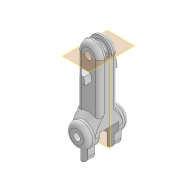
# Autodesk Inventor part: ring_f2
Saved by Autodesk Inventor 2020.2 (Build 242310000, 310)
## iProperties
Created: 2020-04-08
Part Number: ring_f2
Material: Generic
Document SubType Name: Modeling
Designer: Bardo91
Density: 1 g/cm^3
Appearance: Default
Author: Bardo91
Autodesk Inventor part; units mm, degrees
ref_plane "YZ Plane" through (0, 0, 0) normal (1, 0, 0) x (0, 1, 0)
ref_plane "XY Plane" through (0, 0, 0) normal (0, 0, 1) x (1, 0, 0)
sketch "Sketch1" plane through (0, 0, 0) normal (0, 0, 1) x (1, 0, 0)
  circle A0 centre (0, 0) radius 1.5
  circle A1 centre (0, 0) radius 5
  line L0 (0, 0) -> (0, 28)
  circle A2 centre (0, 28) radius 1.5
  circle A3 centre (0, 28) radius 5
  line L1 (-5, 28) -> (-5, 0)
  line L2 (5, 28) -> (5, 0)
  dimension "d0" = 3
  dimension "d1" = 10
  dimension "d2" = 28
  dimension "d3" = 3
  dimension "d4" = 10
  constraints: 6 end point, 4 centre point, 4 coincident, 4 point on circle, 3 tangent, 1 vertical
  measures "d0" diameter of A0
  measures "d1" diameter of A1
  measures "d2" distance of L0.start L0.end
  measures "d3" diameter of A2
  measures "d4" diameter of A3
extrude "base" add sketch "Sketch1" along normal blind 8
sketch "Sketch2" plane through (0, 0, 8) normal (0, 0, 1) x (1, 0, 0)
  circle A0 centre (0, 0) radius 1.5
  circle A1 centre (0, 0) radius 5
  dimension "d29" = 3.5
  dimension "d7" = 3
  dimension "d8" = 10
  constraints: 2 centre point, 2 coincident
  measures "d7" diameter of A0
  measures "d8" diameter of A1
extrude "joint" add sketch "Sketch2" along normal blind 5
ref_plane "Work Plane1" through (0, 0, 4) normal (0, 0, 1) x (1, 0, 0)
mirror "Mirror1" about plane through (0, 0, 4) normal (0, 0, 1) of "joint"
chamfer "Chamfer1" distance 2 angle 45 2 edges at (0, 5, 8) (0, 5, 0)
sketch "Sketch3" plane through (0, 0, 4) normal (0, 0, 1) x (1, 0, 0)
  circle A0 centre (0, 0) radius 1.5 projected
  circle A1 centre (0, 0) radius 5.25
  line L0 (0, 0) -> (-10, 0)
  line L1 (-10, 0) -> (-10, 5.25)
  line L2 (-10, 5.25) -> (0, 5.25)
  line L3 (0, 0) -> (0, 5.25)
  point P0 (-5.25, 0)
  dimension "d14" = 10.5
  dimension "d21" = 10
  dimension "d22" = 5.25
  constraints: 8 end point, 2 horizontal, 2 perpendicular, 1 coincident, 3 other
  measures "d21" distance of L0.start L0.end
  measures "d22" distance of L0.end L1.end
extrude "joint_2" cut sketch "Sketch3" along normal mid plane 8.5
fillet "Fillet1" radius 2 8 edges at (-5, 0, -5) (0, 33, 0) (-5, 16.625, 0) (5, 16.4495, 0) (0, 33, 8) (-5, 16.625, 8) (5, 16.4495, 8) (-5, 0, 13)
sketch "Sketch5" plane through (0, 0, 0) normal (0, 1, 0) x (-1, 0, 0)
  line L0 (0, -0.25) -> (0, 8.25) projected
  line L1 (0, 4) -> (-3.5, 4)
  line L2 (0, 4) -> (3.5, 4)
  circle A0 centre (-3.5, 4) radius 1.25
  circle A1 centre (3.5, 4) radius 1.25
  point P0 (0, 0)
  dimension "d23" = 3.5
  dimension "d24" = 3.5
  dimension "thread_hole" = 2.5
  dimension "d26" = 2.5
  constraints: 4 end point, 2 centre point, 2 coincident, 2 horizontal, 1 midpoint
  measures "d23" distance of L1.start L1.end
  measures "d24" distance of L1.start L2.end
  measures "thread_hole" diameter of A0
  measures "d26" diameter of A1
extrude "thread_hole" cut sketch "Sketch5" along normal through all contours A0
ref_plane "Work Plane2" through (5, 28, 2) normal (0, 1, 0) x (-1, 0, 0)
sketch "Sketch6" plane through (5, 28, 2) normal (0, 1, 0) x (-1, 0, 0)
  line L0 (5, -2.25) -> (5, 6.25) projected
  line L1 (5, 2) -> (1.5, 2)
  circle A0 centre (1.5, 2) radius 1.25
  line L2 (1.5, 0.75) -> (0, 0.75)
  line L3 (0, 4) -> (0, 0) projected
  line L4 (1.5, 3.25) -> (0, 3.25)
  line L5 (0, 3.25) -> (0, 0.75)
  point P0 (5, -2)
  point P1 (0, 3.25)
  dimension "d29" = 3.5
  dimension "d30" = 2.5
  constraints: 8 end point, 2 horizontal, 2 point on circle, 1 centre point, 1 coincident, 1 midpoint, 1 parallel, 1 perpendicular, 1 point on line, 1 tangent
  measures "d29" distance of L1.start L1.end
  measures "d30" diameter of A0
revolve "thread_hole_end" cut sketch "Sketch6" angle 180 about axis through (0, 28, -0.25) along (0, 0, 1)
sketch "Sketch8" plane through (0, 0, 8.25) normal (0, 0, -1) x (-1, 0, 0)
  line L0 (0, 0) -> (0, -5)
  arc A0 (-5, 0) -> (5, 0) centre (0, 0) ccw projected
  line L1 (0, -5) -> (0, -10)
  line L2 (0, -10) -> (-3, -10)
  line L3 (-3, -10) -> (-3, -4)
  dimension "d35" = 5
  dimension "d36" = 3
  constraints: 8 end point, 2 perpendicular, 2 point on circle, 1 point on line, 1 vertical
  measures "d35" distance of L0.end L1.end
  measures "d36" distance of L1.end L2.end
extrude "lock_1" add sketch "Sketch8" against normal blind 3
mirror "Mirror2" about plane through (0, 0, 4) normal (0, 0, 1) of "lock_1"
fillet "Fillet3" radius 3 2 edges at (3, -10, 9.75) (3, -10, -1.75)
sketch "Sketch9" plane through (0, 0, 8) normal (0, 0, 1) x (1, 0, 0)
  circle A0 centre (0, 28) radius 1.5 projected
  line L0 (0, 28) -> (0, 22)
  line L1 (0, 22) -> (0, 19)
  line L2 (0, 28) -> (1.5869, 19)
  line L3 (0, 28) -> (9.1388, 28) construction
  line L4 (1.5869, 19) -> (0, 19)
  line L5 (0, 22) -> (1.058, 22)
  point P0 (0, 0)
  dimension "d41" = 6
  dimension "d42" = 3
  dimension "d43" = 80
  constraints: 12 end point, 2 horizontal, 2 point on line, 1 equal length, 1 parallel, 1 vertical
  measures "d41" distance of L0.start L0.end
  measures "d42" distance of L0.end L1.end
  measures "d43" angle of L2 L3
extrude "lock_2" add sketch "Sketch9" along normal blind 3 contours L5 L2 L4 L1
mirror "Mirror3" about plane through (0, 0, 4) normal (0, 0, 1) of "lock_2"
chamfer "Chamfer2" distance 3 angle 45 2 edges at (0, 20.5, 8) (0, 20.5, 0)
sketch "Sketch10" plane through (0, 0, 4) normal (0, 0, 1) x (1, 0, 0)
  spline S0 degree 2 poles (-3.5, 0) (-2.205, 10.3057) (-5, 13) knots 0 0 0 1 1 1
  line L0 (-5, 13) -> (-7.6096, 13.9801)
  point P0 (0, 0)
  point P1 (-3.5, 10)
  dimension "d49" = 3.5
  dimension "d50" = 10
  dimension "d54" = 3
  constraints: 2 end point, 3 other
  measures "d49" distance of point (0, 0) point (-3.5, 0)
  measures "d50" distance of point (-3.5, 0) point (-3.5, 10)
  measures "d54" vertical distance of L0.start point (-3.5, 10)
sketch "Sketch11" plane through (0, 0, 0) normal (0, 1, 0) x (-1, 0, 0)
  line L0 (0, -0.25) -> (0, 8.25) projected
  line L1 (0, 4) -> (3.5, 4)
  arc A0 (3.5, 5.25) -> (3.5, 2.75) centre (3.5, 4) ccw projected
  circle A1 centre (3.5, 4) radius 1.25
  point P0 (0, 0)
  point P1 (3.5, 5.25)
  dimension "d52" = 3.5
  constraints: 2 end point, 1 coincident, 1 horizontal, 1 midpoint, 3 other
  measures "d52" distance of L1.start L1.end
sweep "Sweep1" cut profiles "Sketch11" path "Sketch10"
equation "\"d26\" = thread_hole"
equation "\"d30\" = thread_hole"
equation "\"d52\" = d49"
body "Solid1"
